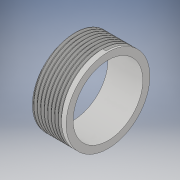
# Autodesk Inventor part: Thread_Metric
Saved by Autodesk Inventor 2019 (Build 230136000, 136)
## iProperties
Created: 2019-04-30
Part Number: Thread_Metric
Material: Generic
Document SubType Name: Modeling
Designer: rhabluet
Density: 1 g/cm^3
Appearance: Default
Author: rhabluet
## iProperties of the stored document Thread_Metric_3DPrint.ipt
Created: 2019-05-01
Part Number: Thread_Metric_3DPrint
Material: Generic
Document SubType Name: Modeling
Designer: rhabluet
Density: 1 g/cm^3
Appearance: Default
Author: rhabluet
Autodesk Inventor part; units mm, degrees
ref_plane "YZ Plane" through (0, 0, 0) normal (1, 0, 0) x (0, 1, 0)
ref_plane "XZ Plane" through (0, 0, 0) normal (0, 1, 0) x (-1, 0, 0)
ref_plane "XY Plane" through (0, 0, 0) normal (0, 0, 1) x (1, 0, 0)
sketch "Sketch2" plane through (0, 0, 0) normal (1, 0, 0) x (0, 1, 0)
  circle A0 centre (0, 0) radius 12
  circle A1 centre (0, 0) radius 10
  dimension "d0" = 24
  dimension "d3" = 20
  constraints: 2 centre point, 2 coincident
  measures "d0" diameter of A0
  measures "d3" diameter of A1
extrude "Extrusion2" add sketch "Sketch2" along normal blind 10
sketch "Sketch3" plane through (0, 0, 0) normal (0, 0, 1) x (1, 0, 0)
  line L0 (0, -16.6859) -> (0, 16.7719) construction
  line L1 (-0.5, 12.1077) -> (-1.5, 12.1077) construction
  line L2 (-1.5, 12.1077) -> (-1.4378, 12) construction
  line L3 (-1.4378, 12) -> (-1.125, 11.4582)
  line L4 (-1.125, 11.4582) -> (-1, 11.2417) construction
  line L5 (-1, 11.2417) -> (-0.875, 11.4582) construction
  line L6 (-0.875, 11.4582) -> (-0.5622, 12)
  line L7 (-0.5622, 12) -> (-0.5, 12.1077) construction
  line L8 (-1.4378, 12) -> (-0.5622, 12)
  line L9 (-1.125, 11.4582) -> (-0.875, 11.4582) construction
  arc A0 (-1.125, 11.4582) -> (-0.875, 11.4582) centre (-1, 11.5303) ccw
  line L10 (0, 12) -> (0, -12) projected
  line L11 (-1, 11.2417) -> (-0.7036, 11.2417) construction
  point P0 (0, 0)
  point P1 (-1, 12)
  dimension "d6" = 60
  dimension "d7" = 1
  dimension "d10" = 60
  dimension "d11" = 1
  dimension "d20" = 0.614
  dimension "d22" = 0.1443
  constraints: 20 end point, 6 point on line, 4 horizontal, 2 point on circle, 2 tangent, 1 centre point, 1 midpoint
  measures "d6" angle of L5 L4
  measures "d7" distance of L1.start L1.end
  measures "d10" angle of L8 L3
  measures "d11" distance of L10.start point (-1, 12)
  measures "d22" distance edge to line of A0 L11
coil "Coil1" sketch "Sketch3" operation cut axis through (-10, 0, 0) along (1, 0, 0) pitch 1 turns 10 hand right
equation "\"d12\" = pitch"
equation "\"d7\" = pitch"
equation "\"d11\" = pitch"
equation "\"d20\" = 0.614 * pitch"
equation "\"d22\" = 0.144333 * pitch"
equation "\"pitch\" = 1"
body "Solid2"
